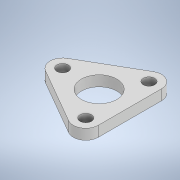
# Autodesk Inventor part: Part2
Saved by Autodesk Inventor 2021 (Build 250183000, 183)
## iProperties
Created: 2022-04-24
Part Number: Part2
Material: Generic
Document SubType Name: Modeling
Designer: hp
Density: 1 g/cm^3
Appearance: Default
Author: hp
Autodesk Inventor part; units mm, degrees
ref_plane "YZ Plane" through (0, 0, 0) normal (1, 0, 0) x (0, 1, 0)
ref_plane "XZ Plane" through (0, 0, 0) normal (0, 1, 0) x (-1, 0, 0)
ref_plane "XY Plane" through (0, 0, 0) normal (0, 0, 1) x (1, 0, 0)
sketch "Sketch1" plane through (0, 0, 0) normal (0, 1, 0) x (-1, 0, 0)
  circle A0 centre (64.977, -75.4393) radius 17
  line L0 (64.977, -75.4393) -> (99.977, -75.4393)
  line L1 (64.977, -75.4393) -> (47.477, -45.1285)
  line L2 (64.977, -75.4393) -> (47.477, -105.7502)
  circle A1 centre (47.477, -45.1285) radius 12
  circle A2 centre (99.977, -75.4393) radius 12
  circle A3 centre (47.477, -105.7502) radius 12
  circle A4 centre (47.477, -45.1285) radius 5.5
  circle A5 centre (99.977, -75.4393) radius 5.5
  circle A6 centre (47.477, -105.7502) radius 5.5
  line L3 (105.977, -65.047) -> (53.477, -34.7362)
  line L4 (35.477, -45.1285) -> (35.477, -105.7502)
  line L5 (53.477, -116.1425) -> (105.977, -85.8317)
  point P0 (0, 0)
  dimension "d0" = 120
  dimension "d1" = 120
  dimension "d2" = 120
  dimension "d3" = 35
  dimension "d5" = 34
  dimension "d6" = 35
  dimension "d7" = 35
  dimension "d8" = 24
  dimension "d9" = 24
  dimension "d10" = 24
  dimension "d11" = 11
  dimension "d13" = 11
  dimension "d14" = 11
  constraints: 12 end point, 7 centre point, 6 coincident, 6 point on circle, 5 tangent, 1 horizontal, 1 vertical
  measures "d0" angle of L2 L0
  measures "d1" angle of L1 L0
  measures "d2" angle of L1 L2
  measures "d3" distance of L0.start L1.end
  measures "d5" diameter of A0
  measures "d6" distance of L0.start L0.end
  measures "d7" distance of L0.start L2.end
  measures "d8" diameter of A1
  measures "d9" diameter of A2
  measures "d10" diameter of A3
  measures "d11" diameter of A4
  measures "d13" diameter of A5
  measures "d14" diameter of A6
extrude "Extrusion1" add sketch "Sketch1" along normal blind 10 contours L0 A2 L5 A3 L2 A0 | A0 L1 A1 L3 A2 L0 | A0 L2 A3 L4 A1 L1 | A2 | A1 | A3
equation "\"d1\" = d0"
equation "\"d6\" = d3"
equation "\"d7\" = d3"
equation "\"d9\" = d8"
equation "\"d10\" = d8"
equation "\"d13\" = d11"
body "Solid1"
